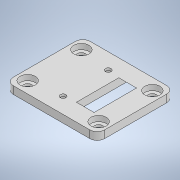
# Autodesk Inventor part: Крепление двигателя2
Saved by Autodesk Inventor 2020 (Build 240168000, 168)
## iProperties
Created: 2021-06-13
Part Number: Крепление двигателя2
Material: Типовые
Document SubType Name: Обычные детали
Designer: Антон
Density: 1 g/cm^3
Appearance: По умолчанию
Author: Антон
Autodesk Inventor part; units mm, degrees
ref_plane "YZ Plane" through (0, 0, 0) normal (1, 0, 0) x (0, 1, 0)
ref_plane "XZ Plane" through (0, 0, 0) normal (0, 1, 0) x (-1, 0, 0)
ref_plane "XY Plane" through (0, 0, 0) normal (0, 0, 1) x (1, 0, 0)
sketch "Эскиз1" plane through (0, 0, 0) normal (0, 1, 0) x (-1, 0, 0)
  line L0 (0, 0) -> (36, 0)
  line L1 (36, 0) -> (36, -30.3)
  line L2 (36, -30.3) -> (0, -30.3)
  line L3 (0, -30.3) -> (0, 0)
  dimension "d0" = 36
  dimension "d1" = 30.3
  constraints: 8 end point, 2 parallel, 1 horizontal, 1 perpendicular
  measures "d0" distance of L1.end L2.end
  measures "d1" distance of L0.end L1.end
extrude "Выдавливание1" add sketch "Эскиз1" along normal blind 3
sketch "Эскиз2" plane through (0, 3, 0) normal (0, 1, 0) x (1, 0, 0)
  line L0 (-36, 30.3) -> (-36, 0) projected
  line L1 (-36, 0) -> (-36, 4.55)
  line L2 (-36, 4.55) -> (-32, 4.55)
  line L3 (-36, 0) -> (0, 0) projected
  line L4 (-18, 0) -> (-18, 30.3)
  line L5 (0, 30.3) -> (-36, 30.3) projected
  line L6 (-36, 15.15) -> (0, 15.15)
  line L7 (0, 0) -> (0, 30.3) projected
  point P0 (-32, 25.75)
  point P1 (-4, 4.55)
  point P2 (-4, 25.75)
  dimension "d4" = 4.55
  dimension "d48" = 4
  constraints: 8 end point, 4 midpoint, 3 symmetric about line, 1 perpendicular, 1 point on line
  measures "d4" distance of L0.end L1.end
  measures "d48" distance of L1.end L2.end
hole "Отверстие1" at (-32, 3, -4.55) at (-32, 3, -25.75) at (-4, 3, -25.75) at (-4, 3, -4.55) direction (0, -1, 0) diameter 3.2 end through all counterbore diameter 6 counterbore depth 2.15
fillet "Сопряжение1" radius 2.95 4 edges at (0, 1.5, 0) (0, 1.5, -30.3) (-36, 1.5, -30.3) (-36, 1.5, 0)
sketch "Эскиз4" plane through (0, 0, -2.95) normal (1, 0, 0) x (0, 0, -1)
  line L0 (12.2, 0) -> (12.2, -13.5)
  circle A0 centre (12.2, -13.5) radius 18.5
  line L1 (0, 0) -> (24.4, 0) projected
  line L2 (0, 0) -> (0, 3) projected
  line L3 (0, 1.5) -> (24.4, 1.5)
  line L4 (24.4, 3) -> (24.4, 0) projected
  dimension "d27" = 13.5
  dimension "d38" = 37
  constraints: 4 end point, 3 midpoint, 1 centre point, 1 coincident, 1 vertical
  measures "d27" distance of L0.start L0.end
  measures "d38" diameter of A0
ref_plane "РабПлоскость1" through (-8, 0, -2.95) normal (1, 0, 0) x (0, 0, -1)
extrude "Выдавливание3" cut sketch "Эскиз4" against normal blind 7 from surface at -8 contours A0 L2 L1 L4 | L4 L1 L2 A0 L3 | L3 A0
sketch "Эскиз6" plane through (0, 3, 0) normal (0, 1, 0) x (1, 0, 0)
  line L0 (-15, 23.5166) -> (-15, 6.7834) projected
  line L1 (-15, 15.15) -> (-19.7, 15.15)
  line L2 (-19.7, 6.25) -> (-19.7, 24.05)
  point P0 (0, 0)
  dimension "d39" = 4.7
  dimension "d40" = 17.8
  constraints: 4 end point, 2 midpoint, 1 horizontal, 1 perpendicular
  measures "d39" distance of L1.end L1.start
  measures "d40" distance of L2.start L2.end
hole "Отверстие2" at (-19.7, 3, -6.25) at (-19.7, 3, -24.05) direction (0, -1, 0) diameter 2.2 end through all
sketch "Эскиз7" plane through (0, 0, 0) normal (0, -1, 0) x (1, 0, 0)
  circle A0 centre (-19.7, -6.25) radius 1.1 projected
  line L0 (-17.3, -7.6356) -> (-19.7, -9.0213)
  line L1 (-19.7, -9.0213) -> (-22.1, -7.6356)
  line L2 (-22.1, -7.6356) -> (-22.1, -4.8644)
  line L3 (-22.1, -4.8644) -> (-19.7, -3.4787)
  line L4 (-19.7, -3.4787) -> (-17.3, -4.8644)
  line L5 (-17.3, -4.8644) -> (-17.3, -7.6356)
  circle A1 centre (-19.7, -24.05) radius 1.1 projected
  line L6 (-17.3, -25.4356) -> (-19.7, -26.8213)
  line L7 (-19.7, -26.8213) -> (-22.1, -25.4356)
  line L8 (-22.1, -25.4356) -> (-22.1, -22.6644)
  line L9 (-22.1, -22.6644) -> (-19.7, -21.2787)
  line L10 (-19.7, -21.2787) -> (-17.3, -22.6644)
  line L11 (-17.3, -22.6644) -> (-17.3, -25.4356)
  line L12 (-15, -2.5009) -> (-15, -27.7991) projected
  point P0 (0, 0)
  dimension "d49" = 4.8
  constraints: 24 end point, 2 coincident, 2 parallel, 1 collinear, 26 other
  measures "d49" distance between parallel lines of L8 L11
extrude "Выдавливание4" cut sketch "Эскиз7" against normal blind 2.1
equation "\"Радиус_гибки\" = Толщина"
equation "\"Ширина_просечки\" = Толщина"
equation "\"Глубина_просечки\" = 0.5 * Толщина"
equation "\"Размер_просечки\" = 4 * Толщина"
equation "\"Мин_остаток\" = 2 * Толщина"
equation "\"Радиус_перехода\" = Радиус_гибки"
equation "\"Радиус_Якоби\" = Толщина"
equation "\"Размер_зазора\" = Толщина"
equation "\"Толщина\" = 0.5"
